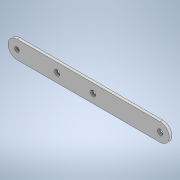
# Autodesk Inventor part: glowny_wahacz
Saved by Autodesk Inventor 2020.3 (Build 243373000, 373)
## iProperties
Created: 2021-10-24
Part Number: glowny_wahacz
Material: Ogólny
Document SubType Name: Modeling
Designer: patry
Density: 1 g/cm^3
Appearance: Domyślna
Author: patry
Autodesk Inventor part; units mm, degrees
ref_plane "YZ Plane" through (0, 0, 0) normal (1, 0, 0) x (0, 1, 0)
ref_plane "XZ Plane" through (0, 0, 0) normal (0, 1, 0) x (-1, 0, 0)
ref_plane "XY Plane" through (0, 0, 0) normal (0, 0, 1) x (1, 0, 0)
sketch "Szkic1" plane through (0, 0, 0) normal (0, 0, 1) x (1, 0, 0)
  line L0 (0, 0) -> (160, 0) construction
  line L1 (0, -10) -> (160, -10)
  line L2 (160, 10) -> (0, 10)
  arc A0 (0, 10) -> (0, -10) centre (0, 0) ccw
  arc A1 (160, -10) -> (160, 10) centre (160, 0) ccw
  point P0 (80, 0)
  point P1 (85, 0)
  point P2 (45, 0)
  dimension "d0" = 160
  dimension "d1" = 20
  dimension "d2" = 75
  dimension "d12" = 45
  constraints: 8 end point, 4 point on circle, 4 tangent, 2 centre point, 2 coincident, 2 point on line, 1 horizontal, 1 midpoint, 1 parallel
  measures "d0" distance of L0.start L0.end
  measures "d1" diameter of A1
  measures "d2" distance of point (160, 0) point (85, 0)
  measures "d12" distance of point (0, 0) point (45, 0)
extrude "Wyciągnięcie proste1" add sketch "Szkic1" along normal blind 3
hole "Otwór1" at (160, 0, 0) at (85, 0, 0) at (45, 0, 0) direction (0, 0, 1) diameter 6 end through all
hole "Otwór2" at (0, 0, 0) direction (0, 0, 1) diameter 5 end through all
